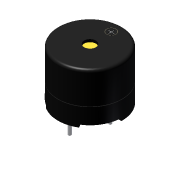
# Autodesk Inventor part: buzzer
Saved by Autodesk Inventor 2012 (Build 160160000, 160)
## iProperties
Created: 2015-04-13
Part Number: buzzer
Material: Default
Document SubType Name: Modeling
Designer: s42851
Density: 1 g/cm^3
Author: s42851
Autodesk Inventor part; units mm, degrees
ref_plane "YZ Plane" through (0, 0, 0) normal (1, 0, 0) x (0, 1, 0)
ref_plane "XZ Plane" through (0, 0, 0) normal (0, 1, 0) x (-1, 0, 0)
ref_plane "XY Plane" through (0, 0, 0) normal (0, 0, 1) x (1, 0, 0)
sketch "Sketch1" plane through (0, 0, 0) normal (0, 0, 1) x (1, 0, 0)
  circle A0 centre (0, 0) radius 6
  dimension "d0" = 12
  constraints: 1 centre point, 1 coincident
  measures "d0" diameter of A0
extrude "Extrusion1" add sketch "Sketch1" along normal blind 9.5
ref_plane "Work Plane1" through (0, 0, 9) normal (0, 0, 1) x (1, 0, 0)
sketch "Sketch2" plane through (0, 0, 9) normal (0, 0, 1) x (1, 0, 0)
  circle A0 centre (0, 0) radius 6 projected
  circle A1 centre (0, 0) radius 4.25
  dimension "d4" = 8.5
  constraints: 1 centre point
  measures "d4" diameter of A1
extrude "Extrusion2" cut sketch "Sketch2" against normal blind 1 contours A1
sketch "Sketch3" plane through (0, 0, 9.5) normal (0, 0, 1) x (1, 0, 0)
  circle A0 centre (0, 0) radius 6 projected
  circle A1 centre (0, 0) radius 1.1
  dimension "d7" = 2.2
  constraints: 1 centre point, 1 coincident
  measures "d7" diameter of A1
extrude "Extrusion3" cut sketch "Sketch3" against normal blind 0.5 contours A1
sketch "Sketch4" plane through (0, 0, 0) normal (0, 0, -1) x (-1, 0, 0)
  circle A0 centre (0, 0) radius 6 projected
  circle A1 centre (0, 0) radius 5.25
  dimension "d10" = 10.5
  constraints: 1 centre point
  measures "d10" diameter of A1
extrude "Extrusion4" cut sketch "Sketch4" against normal blind 0.5 contours A1
fillet "Fillet1" radius 0.5 1 edges at (-6, 0, 9.5)
sketch "Sketch5" plane through (0, 0, 0) normal (0, 0, -1) x (-1, 0, 0)
  circle A0 centre (0, 0) radius 5.25 projected
  circle A1 centre (0, 0) radius 6 projected
  line L0 (2.5416, 4.5938) -> (2.9047, 5.25)
  line L1 (-2.5416, 4.5938) -> (-2.9047, 5.25)
  constraints: 4 end point, 4 point on circle
extrude "Extrusion5" cut sketch "Sketch5" against normal blind 0.5 contours A0 L1 A1 L0 picked at (0.1766, 5.7207)
pattern_circular "Circular Pattern1" count 3 over 360 about axis through (0, 0, 0) along (0, 0, 1) of "Extrusion5"
sketch "Sketch6" plane through (0, 0, 0.5) normal (0, 0, -1) x (-1, 0, 0)
  arc A0 (-5.999, -0.1094) -> (-3.0943, -5.1406) centre (0, 0) ccw projected
  circle A1 centre (0, 3.8) radius 0.3
  dimension "d19" = 0.6
  dimension "d20" = 3.8
  constraints: 1 centre point
  measures "d19" diameter of A1
  measures "d20" distance of A1.centre A0.centre
extrude "Extrusion6" add sketch "Sketch6" along normal blind 6
sketch "Sketch7" plane through (0, 0, 0.5) normal (0, 0, -1) x (-1, 0, 0)
  arc A0 (-2.5416, 4.5938) -> (-5.2491, -0.0957) centre (0, 0) ccw projected
  circle A1 centre (0, -3.8) radius 0.3
  dimension "d23" = 0.6
  dimension "d24" = 3.8
  constraints: 1 centre point
  measures "d23" diameter of A1
  measures "d24" distance of A0.centre A1.centre
extrude "Extrusion7" add sketch "Sketch7" along normal blind 4
chamfer "Chamfer1" distance 0.2 angle 45 2 edges at (0.3, 3.8, -5.5) (0.3, -3.8, -3.5)
sketch "Sketch8" plane through (0, 0, 9.5) normal (0, 0, 1) x (1, 0, 0)
  line L0 (-0.7574, 4.5872) -> (0.6588, 4.5872) construction
  line L1 (0.6588, 4.5872) -> (0.6588, 3.3036) construction
  line L2 (0.6588, 3.3036) -> (-0.7574, 3.3036) construction
  line L3 (-0.7574, 3.3036) -> (-0.7574, 4.5872) construction
  line L4 (0.5858, 3.9175) -> (0.0777, 3.9175)
  line L5 (0.0777, 3.9175) -> (0.0777, 3.4094)
  line L6 (0.0777, 3.4094) -> (-0.09, 3.4094)
  line L7 (-0.09, 3.4094) -> (-0.09, 3.9175)
  line L8 (-0.09, 3.9175) -> (-0.5981, 3.9175)
  line L9 (-0.5981, 3.9175) -> (-0.5981, 4.0791)
  line L10 (-0.5981, 4.0791) -> (-0.09, 4.0791)
  line L11 (-0.09, 4.0791) -> (-0.09, 4.5872)
  line L12 (-0.09, 4.5872) -> (0.0777, 4.5872)
  line L13 (0.0777, 4.5872) -> (0.0777, 4.0791)
  line L14 (0.0777, 4.0791) -> (0.5858, 4.0791)
  line L15 (0.5858, 4.0791) -> (0.5858, 3.9175)
  constraints: 2 other
extrude "Extrusion8" cut sketch "Sketch8" against normal blind 0.1
sketch "Sketch9" plane through (0, 0, 9.5) normal (0, 0, 1) x (1, 0, 0)
  circle A0 centre (0, 3.9983) radius 0.824
  circle A1 centre (0, 3.9983) radius 0.8972
  constraints: 2 centre point
extrude "Extrusion9" cut sketch "Sketch9" against normal blind 0.01
ref_plane "Work Plane2" through (0, 0, 3.5) normal (0, 0, 1) x (1, 0, 0)
sketch "Sketch10" plane through (0, 0, 3.5) normal (0, 0, 1) x (1, 0, 0)
  circle A0 centre (0, 0) radius 6 projected
  circle A1 centre (0, 0) radius 5.75
  dimension "d35" = 11.5
  constraints: 1 centre point
  measures "d35" diameter of A1
extrude "Extrusion10" cut sketch "Sketch10" along normal mid plane 0.1
body "Solid1"
